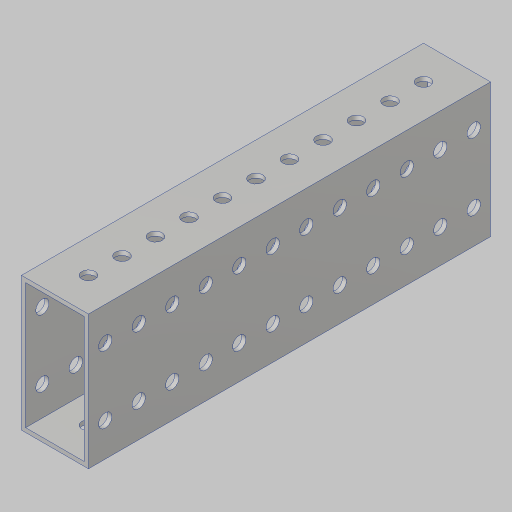
# Autodesk Inventor part: CL7-006
Saved by Autodesk Inventor 2023.5 (Build 275446000, 446)
## iProperties
Created: 2025-03-17
Part Number: CL7-006
Material: Aluminum 6061
Document SubType Name: Modeling
Designer: slick
Mass: 304.185 g
Surface Area: 718.547 cm^2
Volume: 112.661 cm^3
Density: 2.7 g/cm^3
Appearance: Aluminum - Flat
RuleStatus: InUse
AfterDocNew0: SHOW
AfterDocOpen0: SHOW
Author: slick
Autodesk Inventor part; units mm, degrees
ref_plane "YZ Plane" through (0, 0, 0) normal (1, 0, 0) x (0, 1, 0)
ref_plane "XZ Plane" through (0, 0, 0) normal (0, 1, 0) x (-1, 0, 0)
ref_plane "XY Plane" through (0, 0, 0) normal (0, 0, 1) x (1, 0, 0)
sketch "Sketch1" plane through (0, 0, 0) normal (0, 0, 1) x (1, 0, 0)
  line L0 (-12.7, -25.4) -> (12.7, -25.4)
  line L1 (12.7, -25.4) -> (12.7, 25.4)
  line L2 (12.7, 25.4) -> (-12.7, 25.4)
  line L3 (-12.7, 25.4) -> (-12.7, -25.4)
  line L4 (-12.7, -25.4) -> (12.7, 25.4) construction
  line L5 (12.7, -25.4) -> (-12.7, 25.4) construction
  line L6 (-11.1125, 23.8125) -> (11.1125, 23.8125)
  line L7 (11.1125, 23.8125) -> (11.1125, -23.8125)
  line L8 (11.1125, -23.8125) -> (-11.1125, -23.8125)
  line L9 (-11.1125, -23.8125) -> (-11.1125, 23.8125)
  point P0 (0, 0)
  dimension "width" = 25.4
  dimension "height" = 50.8
  dimension "thickness" = 1.5875
  constraints: 20 end point, 4 parallel, 2 midpoint, 2 perpendicular, 1 horizontal, 3 other
  measures "width" distance of L2.end L1.end
  measures "height" distance of L1.end L0.end
  measures "thickness" distance between parallel lines of L2 L6
extrude "Extrusion1" add sketch "Sketch1" along normal mid plane 152.4
sketch "Sketch2" plane through (-12.7, 25.4, 76.2) normal (0, 1, 0) x (1, 0, 0)
  line L0 (25.4, 0) -> (0, 0) construction
  line L1 (0, 152.4) -> (0, 0) construction
  line L2 (25.4, 0) -> (0, 0) construction
  line L3 (25.4, 152.4) -> (25.4, 0) construction
  line L4 (0, 152.4) -> (25.4, 152.4) construction
  point P0 (12.7, 76.2)
  point P1 (12.7, 12.7)
  point P2 (12.7, 25.4)
  point P3 (12.7, 38.1)
  point P4 (12.7, 50.8)
  point P5 (12.7, 63.5)
  point P6 (12.7, 76.2)
  point P7 (12.7, 88.9)
  point P8 (12.7, 101.6)
  point P9 (12.7, 114.3)
  point P10 (12.7, 127)
  point P11 (12.7, 139.7)
  dimension "d5" = 12.7
  dimension "d8" = 12.7
  constraints: 1 vertical, 1 vertical alignment, 10 other
  measures "d5" distance from line of L0 point (12.7, 12.7)
  measures "d8" distance of point (12.7, 12.7) point (12.7, 25.4)
hole "Hole1" at (0, 25.4, 63.5) at (0, 25.4, 50.8) at (0, 25.4, 38.1) at (0, 25.4, 25.4) at (0, 25.4, 12.7) at (0, 25.4, 0) at (0, 25.4, -12.7) at (0, 25.4, -25.4) at (0, 25.4, -38.1) at (0, 25.4, -50.8) at (0, 25.4, -63.5) direction (0, -1, 0) diameter 5.1054 end through all clearance for "Socket Head Cap Screw" size "#10" standard "Ansi Unified Screw Threads"
sketch "Sketch3" plane through (12.7, -25.4, 76.2) normal (1, 0, 0) x (0, 0, -1)
  line L0 (6.35, 38.1) -> (6.35, 12.7) construction
  line L1 (0, 0) -> (0, 50.8) construction
  line L2 (152.4, 50.8) -> (0, 50.8) construction
  line L3 (0, 0) -> (0, 50.8) construction
  line L4 (152.4, 0) -> (0, 0) construction
  line L5 (152.4, 50.8) -> (152.4, 0) construction
  point P0 (76.2, 25.4)
  point P1 (6.35, 25.4)
  point P2 (19.05, 38.1)
  point P3 (19.05, 12.7)
  point P4 (31.75, 38.1)
  point P5 (31.75, 12.7)
  point P6 (44.45, 38.1)
  point P7 (44.45, 12.7)
  point P8 (57.15, 38.1)
  point P9 (57.15, 12.7)
  point P10 (69.85, 38.1)
  point P11 (69.85, 12.7)
  point P12 (82.55, 38.1)
  point P13 (82.55, 12.7)
  point P14 (95.25, 38.1)
  point P15 (95.25, 12.7)
  point P16 (107.95, 38.1)
  point P17 (107.95, 12.7)
  point P18 (120.65, 38.1)
  point P19 (120.65, 12.7)
  point P20 (133.35, 38.1)
  point P21 (133.35, 12.7)
  point P22 (146.05, 38.1)
  point P23 (146.05, 12.7)
  dimension "d20" = 25.4
  dimension "d21" = 6.35
  dimension "d24" = 12.7
  constraints: 2 end point, 1 horizontal, 1 horizontal alignment, 1 midpoint, 1 vertical, 1 vertical alignment, 22 other
  measures "d20" distance of L0.start L0.end
  measures "d21" distance between parallel lines of L1 L0
  measures "d24" distance of L0.start point (19.05, 38.1)
hole "Hole2" at (12.7, 12.7, 69.85) at (12.7, -12.7, 69.85) at (12.7, 12.7, 57.15) at (12.7, -12.7, 57.15) at (12.7, 12.7, 44.45) at (12.7, -12.7, 44.45) at (12.7, 12.7, 31.75) at (12.7, -12.7, 31.75) at (12.7, 12.7, 19.05) at (12.7, -12.7, 19.05) at (12.7, 12.7, 6.35) at (12.7, -12.7, 6.35) at (12.7, 12.7, -6.35) at (12.7, -12.7, -6.35) at (12.7, 12.7, -19.05) at (12.7, -12.7, -19.05) at (12.7, 12.7, -31.75) at (12.7, -12.7, -31.75) at (12.7, 12.7, -44.45) at (12.7, -12.7, -44.45) at (12.7, 12.7, -57.15) at (12.7, -12.7, -57.15) at (12.7, 12.7, -69.85) at (12.7, -12.7, -69.85) direction (-1, 0, 0) diameter 5.1054 end through all clearance for "Socket Head Cap Screw" size "#10" standard "Ansi Unified Screw Threads"
body "Solid1"
